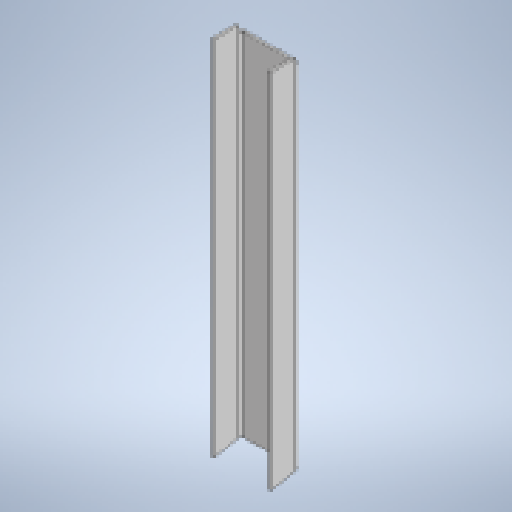
# Autodesk Inventor part: DMF 01 12 wheel pin
Saved by Autodesk Inventor 2025 (Build 290162010, 162A)
## iProperties
Created: 2024-04-30
Part Number: DMF 01 12 wheel pin
Material: Generic
Document SubType Name: Sheet Metal
Designer: admin
Density: 1 g/cm^3
Sheet Metal Rule: Default
Appearance: Default
Sheet Metal Width: 0,000 mm
Sheet Metal Length: 0,000 mm
Sheet Metal Area: 0,000 mm^2
Stock Number: Барабан_Сектор_Усилителя
d50: 0,00 deg
wheel_pin_L: 290,000 mm
wheel_pin_h: 25,000 mm
wheel_pin_Angle: 11,00 deg
Author: pokla
Autodesk Inventor part; units mm, degrees
ref_plane "YZ Plane" through (0, 0, 0) normal (1, 0, 0) x (0, 1, 0)
ref_plane "XZ Plane" through (0, 0, 0) normal (0, 1, 0) x (-1, 0, 0)
ref_plane "XY Plane" through (0, 0, 0) normal (0, 0, 1) x (1, 0, 0)
sketch "Sketch1" plane through (0, 0, 0) normal (0, 0, 1) x (1, 0, 0)
  line L0 (-25, 305) -> (25, 305)
  line L1 (25, 305) -> (25, 0)
  line L2 (25, 0) -> (-25, 0)
  line L3 (-25, 0) -> (-25, 305)
  point P0 (0, 0)
  point P1 (0, 0)
  point P2 (0, 0)
  point P3 (0, 0)
  point P4 (0, 0)
  dimension "d27" = 50
  dimension "d45" = 305
  measures "d27" distance of L1.end L2.end
  measures "d45" distance of L0.end L1.end
extrude "Plate1" add sketch "Sketch1" against normal blind 2
sketch "Sketch2" plane through (-23, 0, -2) normal (-1, 0, 0) x (0, -1, 0)
  line L0 (-305, 0) -> (0, 0)
  line L1 (0, 0) -> (0, 25)
  line L2 (0, 25) -> (-305, 25)
  line L3 (-305, 25) -> (-305, 0)
  constraints: 6 end point, 1 horizontal, 1 perpendicular, 1 vertical
edge flange "Flange1" height 25 angle 90 thickness 2 bend radius 2 thickness toward (-1, 0, 0) relief straight relief width 2 relief depth 1 corner gap 2 corner form 0 edges at (-25, 152.5, 0) (25, 152.5, 0) wall of the first edge with corners at (-23, 305, -2) (-23, 0, -2) (-23, 0, 23) (-23, 305, 23)
bend "Bend1"
corner "Corner1"
sketch "Sketch3" plane through (-25, 0, 23) normal (-1, 0, 0) x (0, 0, 1)
  line L0 (-21, 305) -> (-21, 0)
  line L1 (0, 0) -> (-21, 0)
  line L2 (0, 305) -> (0, 0)
  line L3 (-21, 305) -> (0, 305)
  line L4 (-21, 305) -> (-21, 310)
  line L5 (-21, 310) -> (0, 310)
  line L6 (0, 310) -> (0, 305)
  point P0 (-23, 0)
  dimension "d39" = 5
  measures "d39" distance between parallel lines of L3 L5
sheet face with bend "Face2" sketch "Sketch3" thickness 2 toward (1, 0, 0) bend radius 2 relief straight relief width 2 relief depth 1 contours L4 L5 L6 L3
bend "Bend2"
mirror "Mirror1" about plane through (0, 0, 0) normal (1, 0, 0) of "Face2"
sketch "Sketch4" plane through (-25, 0, 2) normal (-1, 0, 0) x (0, 0, 1)
  line L0 (21, 0) -> (21, 310) projected
  line L1 (21, 10.1405) -> (-4, 15)
  line L2 (-4, 0) -> (-4, 305) projected
  line L3 (0, 0) -> (21, 0) projected
  line L4 (21, 0) -> (-4, 0)
  line L5 (21, 310) -> (0, 310) projected
  point P0 (-2, 0)
  point P1 (0, 0)
  dimension "d46" = 295
  dimension "d48" = 11
  constraints: 4 end point, 2 point on line, 1 collinear
  measures "d46" distance from line of L5 L1.end
  measures "d48" angle of L3 L1
extrude "Extrusion1" cut sketch "Sketch4" along normal through all both and the other way through all
equation "\"d48\" = wheel_pin_Angle"
equation "\"d15\" = Thickness"
equation "\"d29\" = BendReliefWidth"
equation "\"d30\" = BendReliefDepth"
equation "\"d31\" = MinimumRemnant"
equation "\"d32\" = TransitionRadius"
equation "\"d33\" = wheel_pin_h"
equation "\"d35\" = BendRadius"
equation "\"d36\" = CornerReliefSize"
equation "\"d37\" = GapSize"
equation "\"d38\" = JacobiRadiusSize"
equation "\"d40\" = BendRadius"
equation "\"d41\" = BendReliefWidth"
equation "\"d43\" = MinimumRemnant"
equation "\"d42\" = BendReliefDepth"
equation "\"d44\" = TransitionRadius"
equation "\"BendRadius\" = Thickness"
equation "\"BendReliefWidth\" = Thickness"
equation "\"BendReliefDepth\" = 0.5 * Thickness"
equation "\"CornerReliefSize\" = 4 * Thickness"
equation "\"MinimumRemnant\" = 2 * Thickness"
equation "\"TransitionRadius\" = BendRadius"
equation "\"JacobiRadiusSize\" = BendRadius"
equation "\"GapSize\" = Thickness"
equation "\"wheel_pin_L\" = 290"
equation "\"wheel_pin_h\" = 25"
equation "\"wheel_pin_Angle\" = 11deg"
equation "\"Thickness\" = 2"
body "Solid1"
